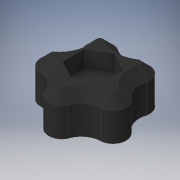
# Autodesk Inventor part: Damper
Saved by Autodesk Inventor 2018 (Build 220112000, 112)
## iProperties
Created: 2017-10-06
Part Number: Damper
Material: Gummi, Butyl
Document SubType Name: Modeling
Designer: tillm
Density: 0.12 g/cm^3
Appearance: Gummi - Schwarz
Author: tillm
Autodesk Inventor part; units mm, degrees
ref_plane "YZ Plane" through (0, 0, 0) normal (1, 0, 0) x (0, 1, 0)
ref_plane "XZ Plane" through (0, 0, 0) normal (0, 1, 0) x (-1, 0, 0)
ref_plane "XY Plane" through (0, 0, 0) normal (0, 0, 1) x (1, 0, 0)
sketch "Skizze1" plane through (0, 0, 0) normal (0, 0, 1) x (1, 0, 0)
  circle A0 centre (0, 0) radius 10 construction
  circle A1 centre (0, 0) radius 11.5 construction
  circle A2 centre (0, 0) radius 8.5 construction
  line L0 (10, 0) -> (8.0902, -5.8779) construction
  line L1 (8.0902, -5.8779) -> (3.0902, -9.5106) construction
  line L2 (3.0902, -9.5106) -> (-3.0902, -9.5106) construction
  line L3 (-3.0902, -9.5106) -> (-8.0902, -5.8779) construction
  line L4 (-8.0902, -5.8779) -> (-10, 0) construction
  line L5 (-10, 0) -> (-8.0902, 5.8779) construction
  line L6 (-8.0902, 5.8779) -> (-3.0902, 9.5106) construction
  line L7 (-3.0902, 9.5106) -> (3.0902, 9.5106) construction
  line L8 (3.0902, 9.5106) -> (8.0902, 5.8779) construction
  line L9 (8.0902, 5.8779) -> (10, 0) construction
  arc A3 (8.0902, 5.8779) -> (10, 0) centre (13.0579, 4.2428) ccw
  arc A4 (8.0902, 5.8779) -> (3.0902, 9.5106) centre (4.7642, 6.5573) ccw
  arc A5 (-3.0902, 9.5106) -> (3.0902, 9.5106) centre (0, 13.7299) ccw
  arc A6 (-3.0902, 9.5106) -> (-8.0902, 5.8779) centre (-4.7642, 6.5573) ccw
  arc A7 (-10, 0) -> (-8.0902, 5.8779) centre (-13.0579, 4.2428) ccw
  arc A8 (-10, 0) -> (-8.0902, -5.8779) centre (-7.7086, -2.5047) ccw
  arc A9 (-3.0902, -9.5106) -> (-8.0902, -5.8779) centre (-8.0703, -11.1078) ccw
  arc A10 (-3.0902, -9.5106) -> (3.0902, -9.5106) centre (0, -8.1053) ccw
  arc A11 (8.0902, -5.8779) -> (3.0902, -9.5106) centre (8.0703, -11.1078) ccw
  arc A12 (8.0902, -5.8779) -> (10, 0) centre (7.7086, -2.5047) ccw
  point P0 (0, -11.5)
  point P1 (10.9371, -3.5537)
  point P2 (6.7595, 9.3037)
  point P3 (-6.7595, 9.3037)
  point P4 (-10.9371, -3.5537)
  dimension "d0" = 20
  dimension "d1" = 23
  dimension "d2" = 17
  constraints: 30 point on circle, 20 end point, 12 centre point, 5 tangent, 4 coincident, 1 horizontal alignment, 23 other
  measures "d1" diameter of A1
  measures "d2" diameter of A2
extrude "Extrusion1" add sketch "Skizze1" along normal blind 10
sketch "Skizze2" plane through (0, 0, 10) normal (0, 0, 1) x (1, 0, 0)
  circle A0 centre (0, 0) radius 5.75 construction
  line L0 (0, 5.75) -> (4.9796, 2.875)
  line L1 (4.9796, 2.875) -> (4.9796, -2.875)
  line L2 (4.9796, -2.875) -> (0, -5.75)
  line L3 (0, -5.75) -> (-4.9796, -2.875)
  line L4 (-4.9796, -2.875) -> (-4.9796, 2.875)
  line L5 (-4.9796, 2.875) -> (0, 5.75)
  dimension "d11" = 11.5
  constraints: 12 end point, 1 coincident, 1 vertical alignment, 15 other
extrude "Extrusion2" cut sketch "Skizze2" against normal blind 4.5
chamfer "Fase1" distance 2.5 angle 45 10 edges at (-8.084, 2.6266, 10) (-10.9371, -3.5537, 10) (-4.9962, -6.8766, 10) (0, -11.5, 10) (4.9962, -6.8766, 10) (10.9371, -3.5537, 10) (8.084, 2.6266, 10) (6.7595, 9.3037, 10) (0, 8.5, 10) (-6.7595, 9.3037, 10)
